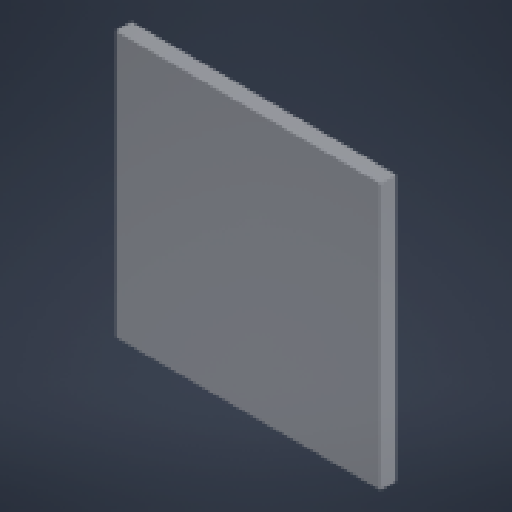
# Autodesk Inventor part: light balance panel
Saved by Autodesk Inventor 2024 (Build 280153000, 153)
## iProperties
Created: 2023-07-17
Part Number: light balance panel
Material: 폴리카보네이트, 흐릿
Document SubType Name: Modeling
Designer: wodyd
Mass: 4.5 g
Surface Area: 53 cm^2
Volume: 3.75 cm^3
Density: 1.2 g/cm^3
Appearance: 폴리카보네이트 - 흐릿함
Author: wodyd
Autodesk Inventor part; units mm, degrees
ref_plane "YZ Plane" through (0, 0, 0) normal (1, 0, 0) x (0, 1, 0)
ref_plane "XZ Plane" through (0, 0, 0) normal (0, 1, 0) x (-1, 0, 0)
ref_plane "XY Plane" through (0, 0, 0) normal (0, 0, 1) x (1, 0, 0)
sketch "스케치1" plane through (0, 0, 0) normal (0, 0, 1) x (1, 0, 0)
  spline S0 degree 3 poles (-15.2612, 12.2515) (-15.0349, 12.6853) (-14.7773, 13.0995) (-14.1966, 13.8896) (-13.8767, 14.2608) (-13.5293, 14.6082) knots 0 0 0 0 0.146771 0.146771 0.294159 0.294159 0.294159 0.294159 projected
  spline S1 degree 3 poles (-13.5293, 14.6082) (-12.7858, 15.269) (-11.9543, 15.7905) (-10.0862, 16.4947) (-9.1079, 16.6525) (-8.1062, 16.6525) knots 0 0 0 0 0.298403 0.298403 0.598924 0.598924 0.598924 0.598924 projected
  spline S2 degree 3 poles (-8.1062, 16.6525) (-7.8174, 16.6525) (-7.4546, 16.5866) (-6.0853, 16.2679) (-4.6907, 15.7628) (-3.4781, 15.2896) knots 0 0 0 0 0.086646 0.086646 0.355547 0.355547 0.355547 0.355547 projected
  spline S3 degree 3 poles (-3.4781, 15.2896) (-3.0595, 15.1088) (-2.6263, 14.9744) (-1.7181, 14.7928) (-1.251, 14.7501) (-0.7808, 14.7501) knots 0 0 0 0 0.136804 0.136804 0.277858 0.277858 0.277858 0.277858 projected
  spline S4 degree 3 poles (-0.7808, 14.7501) (-0.2535, 14.7501) (0.2623, 14.8303) (1.303, 15.1483) (1.8095, 15.3907) (2.2856, 15.6871) knots 0 0 0 0 0.158207 0.158207 0.326474 0.326474 0.326474 0.326474 projected
  spline S5 degree 3 poles (2.2856, 15.6871) (2.9288, 16.0087) (3.6007, 16.2501) (5.0201, 16.5762) (5.7506, 16.6525) (6.4878, 16.6525) knots 0 0 0 0 0.215721 0.215721 0.436896 0.436896 0.436896 0.436896 projected
  spline S6 degree 3 poles (6.4878, 16.6525) (7.6071, 16.6525) (8.6949, 16.4618) (10.6935, 15.6306) (11.5456, 15.0481) (13.3013, 13.3619) (14.0851, 12.1924) (15.1097, 10.2166) (15.4749, 9.2195) (15.9708, 7.0914) (16.0846, 5.9844) (16.0846, 4.8694) knots 0 0 0 0 0.335788 0.335788 0.649311 0.649311 1.066042 1.066042 1.451922 1.451922 1.854033 1.854033 1.854033 1.854033 projected
  spline S7 degree 3 poles (16.0846, 4.8694) (16.0846, 1.2737) (15.262, -1.6239) (13.7487, -5.2119) (13.0412, -6.5055) (11.3461, -8.9093) (10.3819, -9.9944) (9.2987, -10.9739) knots 0 0 0 0 1.078698 1.078698 1.740738 1.740738 2.393565 2.393565 2.393565 2.393565 projected
  spline S8 degree 3 poles (9.2987, -10.9739) (8.6408, -11.5123) (7.9124, -11.9898) (6.441, -12.5997) (5.7252, -12.7627) (4.983, -12.7627) knots 0 0 0 0 0.255029 0.255029 0.477554 0.477554 0.477554 0.477554 projected
  spline S9 degree 3 poles (4.983, -12.7627) (4.7166, -12.7627) (4.3828, -12.7076) (3.6318, -12.548) (3.1427, -12.4109) (2.7115, -12.28) knots 0 0 0 0 0.079924 0.079924 0.194635 0.194635 0.194635 0.194635 projected
  spline S10 degree 3 poles (2.7115, -12.28) (2.0298, -12.0117) (1.2048, -11.7033) (-0.0514, -11.3285) (-0.507, -11.2295) (-0.8092, -11.2295) knots 0 0 0 0 0.219794 0.219794 0.390034 0.390034 0.390034 0.390034 projected
  spline S11 degree 3 poles (-0.8092, -11.2295) (-1.2512, -11.2295) (-1.6961, -11.3049) (-2.6346, -11.5608) (-3.1422, -11.7657) (-3.6201, -11.9961) knots 0 0 0 0 0.132605 0.132605 0.291964 0.291964 0.291964 0.291964 projected
  spline S12 degree 3 poles (-3.6201, -11.9961) (-4.1877, -12.2144) (-4.7785, -12.4014) (-5.8876, -12.6383) (-6.4161, -12.7059) (-6.9421, -12.7059) knots 0 0 0 0 0.182429 0.182429 0.340129 0.340129 0.340129 0.340129 projected
  spline S13 degree 3 poles (-6.9421, -12.7059) (-7.583, -12.7059) (-8.2269, -12.6367) (-9.4043, -12.3085) (-9.9285, -12.0719) (-10.406, -11.7406) knots 0 0 0 0 0.19228 0.19228 0.366605 0.366605 0.366605 0.366605 projected
  spline S14 degree 3 poles (-10.406, -11.7406) (-11.3282, -11.095) (-12.1404, -10.2239) (-13.3474, -8.6615) (-15.2026, -6.1963) (-16.0846, -3.1091) knots 0 0 0 0 0.337694 0.337694 0.593302 0.593302 0.593302 0.593302 projected
  spline S15 degree 3 poles (-16.0846, -3.1091) (-15.3337, -2.9076) (-14.6504, -2.5696) (-13.3763, -1.5844) (-12.8358, -0.9478) (-12.0681, 0.2628) (-11.581, 1.1192) (-10.9842, 3.1586) (-10.8603, 4.0622) (-10.8603, 4.9829) knots 0 0 0 0 0.233256 0.233256 0.483187 0.483187 0.663407 0.663407 0.801191 0.801191 0.801191 0.801191 projected
  spline S16 degree 3 poles (-10.8603, 4.9829) (-10.8603, 5.9854) (-11.0649, 6.9594) (-11.6695, 8.5595) (-12.1993, 9.748) (-13.3408, 11.0751) (-13.6879, 11.3995) (-14.4443, 11.9206) (-14.8379, 12.1168) (-15.2612, 12.2515) knots 0 0 0 0 0.300754 0.300754 0.513178 0.513178 0.592098 0.592098 0.66603 0.66603 0.66603 0.66603 projected
  spline S17 degree 3 poles (0.1846, 16.3969) (-0.7291, 16.3969) (-1.6096, 16.5658) (-2.9769, 17.1375) (-3.4678, 17.4198) (-4.4245, 18.1139) (-4.8791, 18.5298) (-5.2953, 18.9807) knots 0 0 0 0 0.274105 0.274105 0.444593 0.444593 0.628689 0.628689 0.628689 0.628689 projected
  spline S18 degree 3 poles (-5.2953, 18.9807) (-5.9952, 19.8096) (-6.5445, 20.7289) (-7.2862, 22.7782) (-7.4532, 23.8487) (-7.4532, 24.9432) knots 0 0 0 0 0.325461 0.325461 0.65381 0.65381 0.65381 0.65381 projected
  spline S19 degree 3 poles (-7.4532, 24.9432) (-6.4086, 24.7691) (-5.4111, 24.445) (-3.5531, 23.4431) (-2.7409, 22.7941) (-2.0301, 22.0187) knots 0 0 0 0 0.317705 0.317705 0.633268 0.633268 0.633268 0.633268 projected
  spline S20 degree 3 poles (-2.0301, 22.0187) (-1.3509, 21.174) (-0.7665, 20.2451) (-0.0097, 18.3238) (0.1846, 17.3776) (0.1846, 16.3969) knots 0 0 0 0 0.325176 0.325176 0.619265 0.619265 0.619265 0.619265 projected
  line L0 (25, -25) -> (-25, -25) projected
  line L1 (25, 25) -> (25, -25) projected
  line L2 (-25, 25) -> (25, 25) projected
  line L3 (-25, -25) -> (-25, 25) projected
  point P0 (0, 0)
extrude "돌출1" add sketch "스케치1" along normal blind 1.5 contours S0 S1 S2 S3 S4 S5 S6 S7 S8 S9 S10 S11 S12 S13 S14 S15 S16 | S17 S18 S19 S20 | L0 L3 L2 L1
